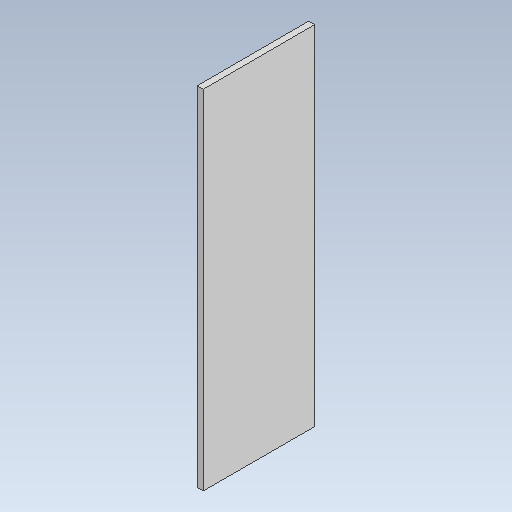
# Autodesk Inventor part: Part2
Saved by Autodesk Inventor 2020.2 (Build 242310000, 310)
## iProperties
Created: 2022-11-14
Part Number: Part2
Material: 一般
Document SubType Name: Modeling
Designer: Administrator
Density: 1 g/cm^3
Appearance: 既定
Author: Administrator
Autodesk Inventor part; units mm, degrees
ref_plane "YZ Plane" through (0, 0, 0) normal (1, 0, 0) x (0, 1, 0)
ref_plane "XZ Plane" through (0, 0, 0) normal (0, 1, 0) x (-1, 0, 0)
ref_plane "XY Plane" through (0, 0, 0) normal (0, 0, 1) x (1, 0, 0)
sketch "スケッチ1" plane through (0, 0, 0) normal (1, 0, 0) x (0, 1, 0)
  line L0 (-30.4084, -19.0054) -> (-20.8087, -18.523) projected
  line L1 (-3.8325, -61.445) -> (-30.2876, -62.7743) projected
  line L2 (83.8546, -57.039) -> (74.2549, -57.5213) projected
  line L3 (57.298, -15.0415) -> (84.0537, -13.6971) projected
  line L4 (85.0253, -13.4226) -> (85.1438, -56.3957) projected
  line L5 (-30.2705, -62.4206) -> (-30.3891, -19.4475) projected
  line L6 (85.1438, -56.3957) -> (-30.3891, -56.3957)
  line L7 (-30.3891, -56.3957) -> (-30.3891, -19.4475)
  line L8 (-30.3891, -19.4475) -> (85.1438, -19.4475)
  line L9 (85.1438, -19.4475) -> (85.1438, -56.3957)
  point P0 (-30.2872, -56.3957)
  point P1 (85.0419, -19.4475)
  point P2 (91.25, 11.0629)
  point P3 (66.1927, -41.4702)
  point P4 (95.1556, -3.15)
  point P5 (65.6556, -3.15)
  point P6 (95.1451, -3.15)
  point P7 (65.6451, -3.15)
  point P8 (94.6925, -3.15)
  point P9 (65.1925, -3.15)
  point P10 (94.6803, -3.15)
  point P11 (65.1803, -3.15)
  constraints: 8 end point, 2 parallel, 1 horizontal, 1 perpendicular
extrude "押し出し1" add sketch "スケッチ1" along normal blind 2 contours L4 L6 L5 L8 | L5 L6 L7
